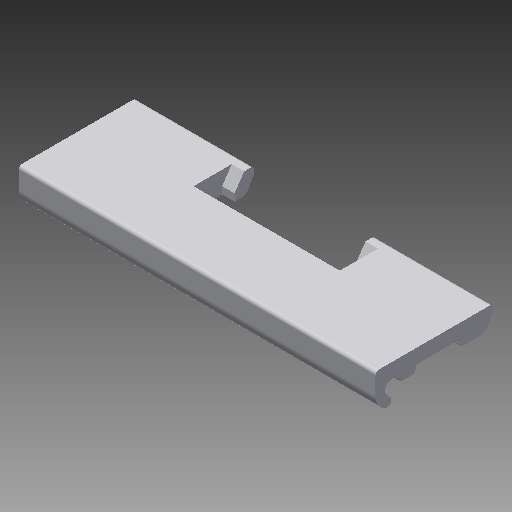
# Autodesk Inventor part: ESG 6.6x20 BHZ 1082540000
Saved by Autodesk Inventor 2019.3 (Build 233278000, 278)
## iProperties
Category: PARTsolutions
Company: WEIDMUELLER
Created: 2018-11-15
Part Number: ESG 6.6x20 BHZ 1082540000
Material: Generic
Catalog Web Link: www.cadenas.de
Description: ESG 6.6x20 BHZ-Elektronikgehäuse
Vendor: WEIDMUELLER
Document SubType Name: Modeling
Designer: psadmin
Manufacturer: WEIDMUELLER
Mass: 0.118333 g
Surface Area: 3.33929 cm^2
Volume: 0.118333 cm^3
Density: 1 g/cm^3
Appearance: PSOLRGB-255-255-255
PSOL_IDENT_0: {$CADENAS_DATA\23d-libs\weidmueller\elektronikgehaeuse\einbaugehaeuse\ch20m\zubehoer\esg_6-6x20_bhz.
PSOL_IDENT_1: prj},198 {VTYP=3D},{NB=ESG 6.6x20 BHZ 1082540000},{LINA=ESG 6.6x20 BHZ 1082540000},{NN=ESG 6.6x20 BH
PSOL_IDENT_2: Z},{DATE=31.03.2017 09:22:39},{GEOMDATE=23.06.2010 00:00:00},{VERSION=},{LINEID=10},{WBVAR=},{WBNUME
PSOL_IDENT_3: RIC=}  {NB=ESG 6.6x20 BHZ 1082540000},{LINA=ESG 6.6x20 BHZ 1082540000},{KT=DUMMY},{BEST=1082540000},
PSOL_IDENT_4: {BZ=ESG 6.6x20 BHZ},{FCODE=1.00,1.00,1.00,0.00}
NN: ESG 6.6x20 BHZ
NT: Elektronikgehäuse
NB: ESG 6.6x20 BHZ 1082540000
NBSYN: $BZ. $BEST.
LINA: ESG 6.6x20 BHZ 1082540000
BEST: 1082540000
BZ: ESG 6.6x20 BHZ
SUPPLIER: WEIDMUELLER
ARTICLENO: ESG 6.6x20 BHZ 1082540000
BOMINFO: ESG 6.6x20 BHZ 1082540000
CREATOR: CADENAS GmbH
Title: ESG 6.6x20 BHZ 1082540000
Author: Cadenas PARTsolutions
Comments: Elektronikgehäuse
Autodesk Inventor part; units mm, degrees
sketch "Sketch_1" plane through (0, 0, 0) normal (1, 0, 0) x (0, 1, 0)
  line L0 (-0.2, 0) -> (-1.2, 0)
  arc A0 (-1.2, 0) -> (-2.0731, -0.5918) centre (-1.2, -0.94) ccw
  arc A1 (-2.0731, -0.5918) -> (-1.6536, -0.8272) centre (-1.83, -0.65) ccw
  line L1 (-1.6536, -0.8272) -> (-1.4822, -0.6565)
  arc A2 (-1.0667, -1.3171) -> (-1.4822, -0.6565) centre (-1.2, -0.94) ccw
  arc A3 (-1.0667, -1.3171) -> (-1.2, -1.5057) centre (-1, -1.5057) ccw
  line L2 (-1.2, -1.5057) -> (-1.2, -2.1)
  arc A4 (-1.2, -2.1) -> (-1.05, -2.25) centre (-1.05, -2.1) ccw
  line L3 (-1.05, -2.25) -> (-0.95, -2.25)
  arc A5 (-0.8, -2.4) -> (-0.95, -2.25) centre (-0.95, -2.4) ccw
  line L4 (-0.8, -2.4) -> (-0.8, -4.6)
  arc A6 (-0.95, -4.75) -> (-0.8, -4.6) centre (-0.95, -4.6) ccw
  line L5 (-0.95, -4.75) -> (-1.05, -4.75)
  arc A7 (-1.05, -4.75) -> (-1.2, -4.9) centre (-1.05, -4.9) ccw
  line L6 (-1.2, -4.9) -> (-1.2, -5.8494)
  arc A8 (-1.2, -5.8494) -> (-0.95, -6.2825) centre (-0.7, -5.8494) ccw
  line L7 (-0.95, -6.2825) -> (-0.4, -6.6)
  line L8 (-0.4, -6.6) -> (-0.2, -6.6)
  arc A9 (-0.2, -6.6) -> (0, -6.4) centre (-0.2, -6.4) ccw
  line L9 (0, -6.4) -> (0, -0.2)
  arc A10 (0, -0.2) -> (-0.2, 0) centre (-0.2, -0.2) ccw
  constraints: 22 point on circle, 20 end point, 11 centre point
extrude "Extrusion1" add sketch "Sketch_1" along normal mid plane 20
sketch "Sketch_2" plane through (0, 0, 0) normal (0, 1, 0) x (-1, 0, 0)
  line L0 (4.1, -3.9) -> (-4.1, -3.9)
  line L1 (-4.1, -3.9) -> (-4.1, -5.5)
  line L2 (-4.1, -5.5) -> (-3.4, -5.5)
  line L3 (-3.4, -5.5) -> (-3.4, -6.9)
  line L4 (-3.4, -6.9) -> (3.4, -6.9)
  line L5 (3.4, -6.9) -> (3.4, -5.5)
  line L6 (3.4, -5.5) -> (4.1, -5.5)
  line L7 (4.1, -5.5) -> (4.1, -3.9)
  constraints: 16 end point
extrude "Extrusion2" cut sketch "Sketch_2" against normal blind 2
sketch "Sketch_4" plane through (0, 0, 0) normal (1, 0, 0) x (0, 1, 0)
  line L0 (0.2, -5.3) -> (-1.0965, -5.3)
  line L1 (-1.0965, -5.3) -> (0.2, -6.1745)
  line L2 (0.2, -6.1745) -> (0.2, -5.3)
  constraints: 6 end point
extrude "Extrusion3" cut sketch "Sketch_4" along normal mid plane 8.2
ref_plane "mitBHZ_XY" through (0, -1.2, -3.9) normal (0, 1, 0) x (1, 0, 0)
ref_plane "mitBHZ_YZ" through (0, -1.2, -3.9) normal (1, 0, 0) x (0, 0, -1)
ref_plane "mitBHZ_ZX" through (0, -1.2, -3.9) normal (0, 0, -1) x (0, 1, 0)
body "Solid1"
